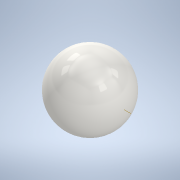
# Autodesk Inventor part: Rueda_Rueda
Saved by Autodesk Inventor 2022.1 (Build 261234000, 234)
## iProperties
Created: 2021-09-10
Part Number: Rueda_Rueda
Material: Genérico
Document SubType Name: Modeling
Designer: seb_0
Density: 1 g/cm^3
Appearance: Acero
Author: seb_0
Autodesk Inventor part; units mm, degrees
ref_plane "YZ Plane" through (0, 0, 0) normal (1, 0, 0) x (0, 1, 0)
ref_plane "XZ Plane" through (0, 0, 0) normal (0, 1, 0) x (-1, 0, 0)
ref_plane "XY Plane" through (0, 0, 0) normal (0, 0, 1) x (1, 0, 0)
sketch "Boceto1" plane through (0, 0, 0) normal (0, 1, 0) x (-1, 0, 0)
  arc A0 (-15, 0) -> (15, 0) centre (0, 0) ccw
  line L0 (0, 0) -> (15, 0)
  line L1 (0, 0) -> (-15, 0)
  line L2 (21, 0) -> (-21, 0) projected
  dimension "d1" = 15
  constraints: 4 end point, 2 horizontal, 2 point on circle, 1 centre point
  measures "d1" radius of A0
revolve "Revolución1" add sketch "Boceto1" angle 360 about axis through (-10, 0, 0) along (1, 0, 0)
